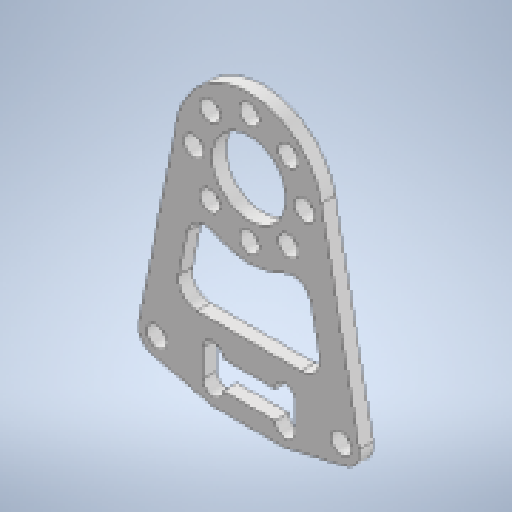
# Autodesk Inventor part: mataroll
Saved by Autodesk Inventor 2025.1 (Build 291241000, 241)
## iProperties
Created: 2024-09-02
Part Number: mataroll
Material: アルミニウム 2014-T4
Document SubType Name: Modeling
Designer: right
Density: 2.8 g/cm^3
Appearance: サテン
Mass: 1.41604 g
Surface Area: 10.7117 cm^2
Volume: 0.50573 cm^3
Author: right
Autodesk Inventor part; units mm, degrees
ref_plane "YZ Plane" through (0, 0, 0) normal (1, 0, 0) x (0, 1, 0)
ref_plane "XZ Plane" through (0, 0, 0) normal (0, 1, 0) x (-1, 0, 0)
ref_plane "XY Plane" through (0, 0, 0) normal (0, 0, 1) x (1, 0, 0)
sketch "スケッチ1" plane through (0, 0, 0) normal (0, 0, 1) x (1, 0, 0)
  circle A0 centre (0, 0) radius 4
  circle A1 centre (0, 0) radius 8
  circle A2 centre (0, 0) radius 6 construction
  circle A3 centre (0, 6) radius 1.1
  circle A4 centre (-4.2426, 4.2426) radius 1.1
  circle A5 centre (-6, 0) radius 1.1
  circle A6 centre (-4.2426, -4.2426) radius 1.1
  circle A7 centre (0, -6) radius 1.1
  circle A8 centre (4.2426, -4.2426) radius 1.1
  circle A9 centre (6, 0) radius 1.1
  circle A10 centre (4.2426, 4.2426) radius 1.1
  arc A11 (8.483, -10.1137) -> (9.4351, -9.068) centre (8.4362, -9.1148) ccw projected
  circle A12 centre (0, 0) radius 13.4197 construction
  circle A13 centre (0, 0) radius 19.4197 construction
  line L0 (5, -19.4197) -> (-5, -19.4197)
  line L1 (-5, -19.4197) -> (-5, -22.4197)
  line L2 (-5, -22.4197) -> (5, -22.4197)
  line L3 (5, -22.4197) -> (5, -19.4197)
  circle A14 centre (3.9, -19.4197) radius 1.1
  line L4 (0, -19.4197) -> (0, -22.4197) construction
  line L5 (0, -20.9197) -> (5, -20.9197) construction
  circle A15 centre (3.9, -22.4197) radius 1.1
  circle A16 centre (-3.9, -19.4197) radius 1.1
  circle A17 centre (-3.9, -22.4197) radius 1.1
  circle A18 centre (10, -20.9197) radius 1.1
  circle A19 centre (-10, -20.9197) radius 1.1
  circle A20 centre (10, -20.9197) radius 2
  circle A21 centre (-10, -20.9197) radius 2
  line L6 (11.9662, -20.5535) -> (7.8647, 1.465)
  line L7 (-11.9662, -20.5535) -> (-7.8647, 1.465)
  circle A22 centre (3.9, -22.4197) radius 2
  circle A23 centre (-3.9, -22.4197) radius 2
  line L8 (3.9, -24.4197) -> (-3.9, -24.4197)
  line L9 (-3.9, -24.4197) -> (-10.4609, -22.8659)
  line L10 (3.9, -24.4197) -> (10.4609, -22.8659)
  point P0 (-5, -19.4197)
  point P1 (-2.8, -19.4197)
  point P2 (2.8, -19.4197)
  point P3 (5, -22.4197)
  point P4 (2.8, -22.4197)
  point P5 (-5, -22.4197)
  point P6 (-5, -22.4197)
  point P7 (-7.8647, 1.465)
  point P8 (-11.9662, -20.5535)
  point P9 (-2.8, -22.4197)
  dimension "d1" = 16
  dimension "d2" = 12
  dimension "d13" = 2.2
  dimension "d17" = 4
  dimension "d18" = 4
  dimension "d19" = 4
  dimension "d0" = 8
  dimension "d3" = 2.2
  dimension "d6" = 360
  dimension "d10" = 6
  dimension "d11" = 10
  dimension "d12" = 3
  dimension "d14" = 2.2
  dimension "d15" = 5
  dimension "d16" = 4
  constraints: 22 end point, 17 centre point, 8 coincident, 6 symmetric about line, 5 vertical alignment, 4 midpoint, 4 tangent, 3 horizontal, 2 parallel, 2 point on circle, 1 horizontal alignment, 1 perpendicular, 1 point on line, 38 other
  measures "d0" diameter of A0
  measures "d3" diameter of A3
  measures "d10" radial gap between concentric circles of A12 A13
  measures "d11" distance of L1.end L2.end
  measures "d12" distance of L0.end L1.end
  measures "d14" diameter of A18
  measures "d15" distance from line of L3 A18.centre
  measures "d16" diameter of A20
extrude "押し出し1" add sketch "スケッチ1" along normal blind 1.5 contours A1 | A1 L6 A20 L10 A22 L3 A14 L0 A16 L1 A23 L9 A21 L7 | A20 | A21 | L10 A22 L2 A15 L3 | A23 L1 A17 L2 L9 | L8 A23 L2 A22
sketch "スケッチ2" plane through (0, 0, 0) normal (0, 0, -1) x (-1, 0, 0)
  circle A0 centre (0, 0) radius 8
  arc A1 (7.8647, 1.465) -> (-7.8647, 1.465) centre (0, 0) ccw projected
  line L0 (-8.1259, -16.3197) -> (8.1259, -16.3197)
  line L1 (8.1259, -16.3197) -> (6.0591, -5.2238)
  line L2 (-6.0591, -5.2238) -> (-8.1259, -16.3197)
  line L3 (7.8647, 1.465) -> (11.9662, -20.5535) projected
  line L4 (-11.9662, -20.5535) -> (-7.8647, 1.465) projected
  arc A2 (-2.8, -19.4197) -> (-5, -19.4197) centre (-3.9, -19.4197) ccw projected
  point P0 (9.9154, -9.5443)
  point P1 (-3.9, -18.3197)
  dimension "d20" = 3
  dimension "d21" = 3
  dimension "d22" = 2
  constraints: 6 end point, 3 point on circle, 2 parallel, 1 centre point, 1 coincident, 1 concentric, 1 horizontal, 1 midpoint
  measures "d20" distance from line of point (9.915, -9.544) L1
  measures "d21" distance between parallel lines of L4 L2
  measures "d22" distance from line of point (-3.9, -18.32) L0
extrude "押し出し2" cut sketch "スケッチ2" against normal through all contours L1 L0 L2 A0
fillet "フィレット1" radius 2 4 edges at (6.0591, -5.2238, 0.75) (-6.0591, -5.2238, 0.75) (-8.1259, -16.3197, 0.75) (8.1259, -16.3197, 0.75)
equation "\"d21\" = d20"
